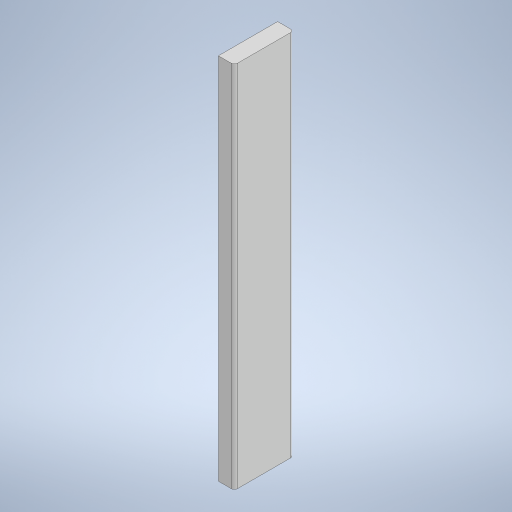
# Autodesk Inventor part: канал_проводов
Saved by Autodesk Inventor 2023.1 (Build 271208000, 208)
## iProperties
Created: 2024-12-20
Part Number: канал_проводов
Material: Типовые
Document SubType Name: Modeling
Designer: DELL
Density: 1 g/cm^3
Appearance: По умолчанию
Author: DELL
Autodesk Inventor part; units mm, degrees
ref_plane "YZ Plane" through (0, 0, 0) normal (1, 0, 0) x (0, 1, 0)
ref_plane "XZ Plane" through (0, 0, 0) normal (0, 1, 0) x (-1, 0, 0)
ref_plane "XY Plane" through (0, 0, 0) normal (0, 0, 1) x (1, 0, 0)
sketch "Эскиз1" plane through (0, 0, 0) normal (0, 1, 0) x (-1, 0, 0)
  line L0 (5, 18.5) -> (-5, 18.5)
  line L1 (-5, 18.5) -> (-5, -18.5)
  line L2 (-5, -18.5) -> (5, -18.5)
  line L3 (5, -18.5) -> (5, 18.5)
  line L4 (5, 18.5) -> (-5, -18.5) construction
  line L5 (-5, 18.5) -> (5, -18.5) construction
  point P0 (0, 0)
  dimension "d0" = 10
  dimension "d1" = 37
  constraints: 12 end point, 2 midpoint, 2 parallel, 1 horizontal, 1 perpendicular
  measures "d0" distance of L2.end L1.end
  measures "d1" distance of L1.end L0.end
extrude "Выдавливание1" add sketch "Эскиз1" along normal blind 230
fillet "Сопряжение1" radius 2 2 edges at (5, 115, 18.5) (5, 115, -18.5)
